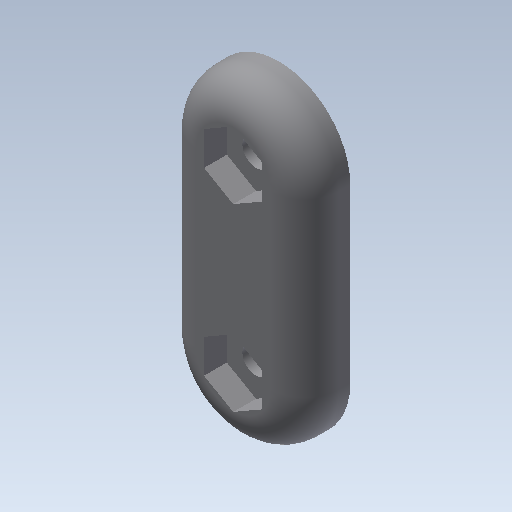
# Autodesk Inventor part: Standard
Saved by Autodesk Inventor 2020.5 (Build 245400000, 400)
## iProperties
RuleStatus: InUse
AfterDocSave0: file://Part Number Cleaner
Created: 2022-05-31
Material: Generic
Catalog Web Link: https://www.janelia.org/
Vendor: HHMI: JRC - jET
Document SubType Name: Modeling
Designer: goulett
Density: 1 g/cm^3
Appearance: Default
LAB/DEPT: A. LEE (LAB)
DESIGN DEPARTMENT: HHMI: JRC - jET
ALTERED ITEM PART NUMBER: N/A
ALTERED ITEM VENDOR: N/A
ALTERED ITEM DESCRIPTION: N/A
Title: Standard
Author: goulett
Revision Number: 0
Autodesk Inventor part; units mm, degrees
ref_plane "YZ Plane" through (0, 0, 0) normal (1, 0, 0) x (0, 1, 0)
ref_plane "XZ Plane" through (0, 0, 0) normal (0, 1, 0) x (-1, 0, 0)
ref_plane "XY Plane" through (0, 0, 0) normal (0, 0, 1) x (1, 0, 0)
sketch "Sketch1" plane through (0, 0, 0) normal (0, 0, 1) x (1, 0, 0)
  line L0 (0, -9.525) -> (0, 9.525) construction
  line L1 (7.9375, -9.525) -> (7.9375, 9.525)
  line L2 (-7.9375, 9.525) -> (-7.9375, -9.525)
  arc A0 (-7.9375, -9.525) -> (7.9375, -9.525) centre (0, -9.525) ccw
  arc A1 (7.9375, 9.525) -> (-7.9375, 9.525) centre (0, 9.525) ccw
  circle A2 centre (0, 10) radius 1.524
  circle A3 centre (0, -10) radius 1.524
  point P0 (0, 0)
  dimension "d0" = 15.875
  dimension "d1" = 3.048
  dimension "d2" = 3.048
  dimension "d3" = 20
  dimension "d4" = 10
  dimension "d5" = 9.525
  constraints: 8 end point, 4 centre point, 4 point on circle, 4 tangent, 2 point on line, 1 midpoint, 1 parallel, 1 vertical
  measures "d0" diameter of A1
  measures "d1" diameter of A2
  measures "d2" diameter of A3
  measures "d3" distance of A2.centre A3.centre
  measures "d4" distance of point (0, 0) A2.centre
  measures "d5" distance of point (0, 0) L0.end
extrude "Extrusion1" add sketch "Sketch1" along normal blind 5.08
sketch "Sketch2" plane through (0, 0, 5.08) normal (0, 0, 1) x (1, 0, 0)
  circle A0 centre (0, 10) radius 1.524 projected
  circle A1 centre (0, -10) radius 1.524 projected
  line L0 (0, 13.7395) -> (3.2385, 11.8697)
  line L1 (3.2385, 11.8697) -> (3.2385, 8.1302)
  line L2 (3.2385, 8.1302) -> (0, 6.2605)
  line L3 (0, 6.2605) -> (-3.2385, 8.1302)
  line L4 (-3.2385, 8.1302) -> (-3.2385, 11.8697)
  line L5 (-3.2385, 11.8697) -> (0, 13.7395)
  line L6 (0, -6.2605) -> (3.2385, -8.1302)
  line L7 (3.2385, -8.1302) -> (3.2385, -11.8697)
  line L8 (3.2385, -11.8697) -> (0, -13.7395)
  line L9 (0, -13.7395) -> (-3.2385, -11.8697)
  line L10 (-3.2385, -11.8697) -> (-3.2385, -8.1302)
  line L11 (-3.2385, -8.1302) -> (0, -6.2605)
  point P0 (0, 0)
  dimension "d8" = 6.477
  constraints: 24 end point, 2 coincident, 2 collinear, 26 other
  measures "d8" distance between parallel lines of L7 L10
extrude "Extrusion2" cut sketch "Sketch2" against normal blind 2.54
fillet "Fillet1" radius 3.81 4 edges at (0, -17.4625, 5.08) (7.9375, 0, 5.08) (0, 17.4625, 5.08) (-7.9375, 0, 5.08)
equation "\"d4\" = 0.5 * d3"
body "Solid1"
